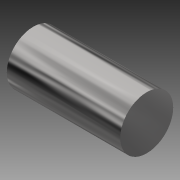
# Autodesk Inventor part: bar
Saved by Autodesk Inventor 2014 (Build 180170000, 170)
## iProperties
Created: 2016-01-12
Part Number: bar
Material: Generic
Document SubType Name: Modeling
Designer: sametj
Density: 1 g/cm^3
Appearance: Default
Author: sametj
Autodesk Inventor part; units mm, degrees
ref_plane "YZ Plane" through (0, 0, 0) normal (1, 0, 0) x (0, 1, 0)
ref_plane "XZ Plane" through (0, 0, 0) normal (0, 1, 0) x (-1, 0, 0)
ref_plane "XY Plane" through (0, 0, 0) normal (0, 0, 1) x (1, 0, 0)
sketch "Sketch1" plane through (0, 0, 0) normal (0, 0, 1) x (1, 0, 0)
  line L0 (382.8474, 31.6164) -> (535.2474, 31.6164)
  line L1 (535.2474, 31.6164) -> (535.2474, -3.9436)
  line L2 (535.2474, -3.9436) -> (382.8474, -3.9436)
  line L3 (382.8474, -3.9436) -> (382.8474, 31.6164)
  line L4 (382.1049, -3.9436) -> (78.4098, -3.9436)
  line L5 (-303.6951, -3.9436) -> (0, 0)
  dimension "d0" = 152.4
  dimension "d1" = 35.56
  dimension "d7" = 303.6951
  dimension "d8" = 303.6951
  constraints: 12 end point, 2 parallel, 1 horizontal, 1 perpendicular
  measures "d0" distance of L1.end L2.end
  measures "d1" distance of L0.end L1.end
  measures "d7" distance of L4.start L4.end
  measures "d8" horizontal distance of L5.start L5.end
revolve "Revolution1" add sketch "Sketch1" angle 360 about axis through (382.8474, 31.6164, 0) along (1, 0, 0)
sketch "Sketch2" plane through (535.2474, 31.6164, 0) normal (1, 0, 0) x (0, 0, -1)
  line L0 (-76.2, 0) -> (76.2, 0)
  point P0 (0, -31.6164)
  constraints: 2 end point, 1 horizontal
revolve "Revolution2" [suppressed]
sketch "Sketch3" plane through (382.8474, 31.6164, 0) normal (-1, 0, 0) x (0, 0, 1)
  line L0 (-76.2, 0) -> (76.2, 0)
  point P0 (0, -31.6164)
  constraints: 2 end point, 1 horizontal
revolve "Revolution3" [suppressed]
body "Solid1"
